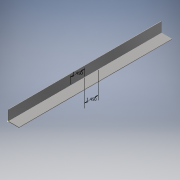
# Autodesk Inventor part: Flywheel Headpiece
Saved by Autodesk Inventor 2017 (Build 210142000, 142)
## iProperties
Created: 2016-10-15
Part Number: Flywheel Headpiece
Material: Steel, Alloy
Document SubType Name: Modeling
Designer: Aditya
Density: 7.73 g/cm^3
Appearance: Semi-Polished
Author: Aditya
Autodesk Inventor part; units mm, degrees
ref_plane "YZ Plane" through (0, 0, 0) normal (1, 0, 0) x (0, 1, 0)
ref_plane "XZ Plane" through (0, 0, 0) normal (0, 1, 0) x (-1, 0, 0)
ref_plane "XY Plane" through (0, 0, 0) normal (0, 0, 1) x (1, 0, 0)
sketch "Sketch1" plane through (0, 0, 0) normal (0, 1, 0) x (-1, 0, 0)
  line L0 (0, 0) -> (0, -406.4)
  line L1 (0, -406.4) -> (27.94, -406.4)
  line L2 (27.94, -406.4) -> (27.94, 0)
  line L3 (27.94, 0) -> (0, 0)
  dimension "d0" = 406.4
  dimension "d1" = 27.94
  constraints: 8 end point, 2 perpendicular, 1 parallel, 1 vertical
  measures "d0" distance of L0.start L0.end
  measures "d1" distance of L0.end L1.end
extrude "Extrusion1" add sketch "Sketch1" along normal blind 1.524
sketch "Sketch2" plane through (0, 0, 0) normal (0, -1, 0) x (1, 0, 0)
  line L0 (-27.94, 0) -> (0, 0) projected
  line L1 (-27.94, 0) -> (-29.464, 0)
  line L2 (-29.464, 0) -> (-29.464, -406.4)
  line L3 (0, -406.4) -> (-27.94, -406.4) projected
  line L4 (-29.464, -406.4) -> (-27.94, -406.4)
  line L5 (-27.94, -406.4) -> (-27.94, 0) projected
  line L6 (-27.94, -406.4) -> (-27.94, 0)
  dimension "d4" = 1.524
  constraints: 8 end point, 3 perpendicular, 1 horizontal
  measures "d4" distance of L0.start L1.end
extrude "Extrusion2" add sketch "Sketch2" against normal blind 27.94
sketch "Sketch3" plane through (-29.464, 0, -406.4) normal (-1, 0, 0) x (0, 0, 1)
  line L0 (406.4, 1.524) -> (0, 1.524) projected
  line L1 (203.2, 1.524) -> (166.37, 1.524)
  line L2 (203.2, 1.524) -> (240.03, 1.524)
  point P0 (406.4, 0)
  dimension "d7" = 36.83
  dimension "d8" = 36.83
  constraints: 4 end point, 2 point on line, 1 midpoint
  measures "d7" distance of L1.start L1.end
  measures "d8" distance of L1.start L2.end
sketch "Sketch4" plane through (-29.464, 0, -406.4) normal (-1, 0, 0) x (0, 0, 1)
  line L0 (0, 1.524) -> (0, 27.94) projected
  line L1 (0, 14.732) -> (406.4, 14.732)
  line L2 (406.4, 1.524) -> (406.4, 27.94) projected
  point P0 (406.4, 0)
  constraints: 2 end point, 2 midpoint
sketch "Sketch5" plane through (-29.464, 0, -406.4) normal (-1, 0, 0) x (0, 0, 1)
  circle A0 centre (250.1934, 14.732) radius 3.937 projected
  circle A1 centre (156.2193, 14.732) radius 3.937 projected
  point P0 (406.4, 0)
extrude "Extrusion3" cut sketch "Sketch5" against normal blind 23.8125
body "Solid1"
